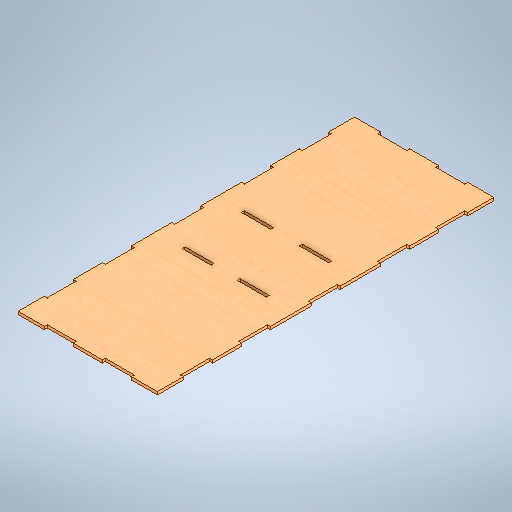
# Autodesk Inventor part: Base
Saved by Autodesk Inventor 2025 (Build 290162000, 162)
## iProperties
Created: 2024-11-02
Part Number: Base
Material: Wood (Cherry)
Document SubType Name: Sheet Metal
Designer: g.marin
Density: 0.63 g/cm^3
Sheet Metal Rule: Default
Appearance: Cherry - Natural Low Gloss
Author: g.marin
Autodesk Inventor part; units mm, degrees
ref_plane "YZ Plane" through (0, 0, 0) normal (1, 0, 0) x (0, 1, 0)
ref_plane "XZ Plane" through (0, 0, 0) normal (0, 1, 0) x (-1, 0, 0)
ref_plane "XY Plane" through (0, 0, 0) normal (0, 0, 1) x (1, 0, 0)
sketch "Sketch1" plane through (0, 0, 0) normal (0, 1, 0) x (-1, 0, 0)
  line L0 (240, 340) -> (0, 340)
  line L1 (0, 340) -> (0, 100)
  line L2 (0, 100) -> (240, 100)
  line L3 (240, 100) -> (240, 340)
  line L4 (240, 0) -> (0, 0)
  line L5 (0, 0) -> (0, -240)
  line L6 (0, -240) -> (240, -240)
  line L7 (240, -240) -> (240, 0)
  line L8 (240, 100) -> (0, 100)
  line L9 (0, 100) -> (0, 0)
  line L10 (0, 0) -> (240, 0)
  line L11 (240, 0) -> (240, 100)
  line L12 (240, 25) -> (235, 25)
  line L13 (235, 25) -> (235, 75)
  line L14 (235, 75) -> (240, 75)
  line L15 (240, 75) -> (240, 25)
  line L16 (240, 145) -> (235, 145)
  line L17 (235, 145) -> (235, 195)
  line L18 (235, 195) -> (240, 195)
  line L19 (240, 195) -> (240, 145)
  line L20 (240, 245) -> (235, 245)
  line L21 (235, 245) -> (235, 295)
  line L22 (235, 295) -> (240, 295)
  line L23 (240, 295) -> (240, 245)
  line L24 (120, -240) -> (120, 340) construction
  line L25 (240, 50) -> (0, 50) construction
  line L26 (240, -45) -> (235, -45)
  line L27 (235, -45) -> (235, -95)
  line L28 (235, -95) -> (240, -95)
  line L29 (240, -145) -> (235, -145)
  line L30 (235, -145) -> (235, -195)
  line L31 (235, -195) -> (240, -195)
  line L32 (0, 25) -> (5, 25)
  line L33 (5, 25) -> (5, 75)
  line L34 (5, 75) -> (0, 75)
  line L35 (0, 145) -> (5, 145)
  line L36 (5, 145) -> (5, 195)
  line L37 (5, 195) -> (0, 195)
  line L38 (0, 245) -> (5, 245)
  line L39 (5, 245) -> (5, 295)
  line L40 (5, 295) -> (0, 295)
  line L41 (5, -45) -> (5, -95)
  line L42 (5, -95) -> (0, -95)
  line L43 (0, -45) -> (5, -45)
  line L44 (5, -195) -> (0, -195)
  line L45 (5, -145) -> (5, -195)
  line L46 (0, -145) -> (5, -145)
  line L47 (195, -240) -> (145, -240)
  line L48 (145, -240) -> (145, -235)
  line L49 (145, -235) -> (195, -235)
  line L50 (195, -235) -> (195, -240)
  line L51 (95, -240) -> (45, -240)
  line L52 (45, -240) -> (45, -235)
  line L53 (45, -235) -> (95, -235)
  line L54 (95, -235) -> (95, -240)
  line L55 (145, 340) -> (145, 335)
  line L56 (145, 335) -> (195, 335)
  line L57 (195, 335) -> (195, 340)
  line L58 (45, 340) -> (45, 335)
  line L59 (45, 335) -> (95, 335)
  line L60 (95, 335) -> (95, 340)
  line L61 (240, -120) -> (0, -120) construction
  line L62 (240, 220) -> (0, 220) construction
  line L63 (145, 0) -> (145, -5)
  line L64 (145, -5) -> (195, -5)
  line L65 (195, -5) -> (195, 0)
  line L66 (45, 0) -> (45, -5)
  line L67 (45, -5) -> (95, -5)
  line L68 (95, -5) -> (95, 0)
  line L69 (192.5, 100) -> (142.5, 100)
  line L70 (142.5, 100) -> (142.5, 105)
  line L71 (142.5, 105) -> (192.5, 105)
  line L72 (192.5, 105) -> (192.5, 100)
  line L73 (97.5, 100) -> (47.5, 100)
  line L74 (47.5, 100) -> (47.5, 105)
  line L75 (47.5, 105) -> (97.5, 105)
  line L76 (97.5, 105) -> (97.5, 100)
  point P0 (240, 0)
  point P1 (237.5, 245)
  point P2 (240, 195)
  point P3 (240, 295)
  point P4 (195, 340)
  point P5 (145, 340)
  point P6 (95, 340)
  point P7 (45, 340)
  point P8 (0, 295)
  point P9 (0, 245)
  point P10 (0, 195)
  point P11 (0, 145)
  point P12 (0, -45)
  point P13 (0, -95)
  point P14 (0, -145)
  point P15 (0, -195)
  point P16 (45, -240)
  point P17 (145, -240)
  point P18 (240, -195)
  point P19 (240, -145)
  point P20 (240, -95)
  point P21 (240, -45)
  point P22 (145, 0)
  point P23 (195, 0)
  point P24 (45, 0)
  point P25 (95, 0)
  point P26 (97.5, 102.5)
  point P27 (142.5, 102.5)
  point P28 (120, 100)
  point P29 (47.5, 100)
  point P30 (97.5, 100)
  point P31 (192.5, 100)
  dimension "d0" = 240
  dimension "d1" = 240
  dimension "d2" = 240
  dimension "d3" = 100
  dimension "d6" = 50
  dimension "d7" = 50
  dimension "d8" = 50
  dimension "d9" = 50
  dimension "d10" = 45
  dimension "d12" = 5
  dimension "d13" = 25
  dimension "d14" = 5
  dimension "d15" = 45
  dimension "d16" = 50
  dimension "d17" = 50
  dimension "d18" = 50
  dimension "d19" = 50
  dimension "d20" = 50
  dimension "d21" = 5
  dimension "d22" = 45
  dimension "d23" = 22.5
  constraints: 154 end point, 44 symmetric about line, 20 parallel, 19 point on line, 12 midpoint, 11 perpendicular, 10 horizontal, 1 coincident
  measures "d0" distance of L2.end L0.start
  measures "d1" distance of L0.start L0.end
  measures "d2" distance of L6.end L4.start
  measures "d3" distance of L10.end L2.end
  measures "d6" distance of L12.end L13.end
  measures "d7" distance of L16.end L17.end
  measures "d8" distance of L20.end L21.end
  measures "d9" distance from line of point (237.5, 245) L18
  measures "d10" distance between parallel lines of L0 L22
  measures "d12" distance between parallel lines of L13 L15
  measures "d13" distance between parallel lines of L12 L4
  measures "d14" distance between parallel lines of L49 L6
  measures "d15" distance between parallel lines of L50 L7
  measures "d16" distance of L48.end L49.end
  measures "d17" distance of L52.end L53.end
  measures "d18" distance between parallel lines of L54 L48
  measures "d19" distance of L70.end L71.end
  measures "d20" distance of L74.end L75.end
  measures "d21" distance of L69.end L70.end
  measures "d22" distance of point (97.5, 102.5) point (142.5, 102.5)
  measures "d23" horizontal distance of point (120, 100) L70.end
extrude "Extrusion1" add sketch "Sketch1" along normal blind 5 contours L3 L22 L21 L20 L18 L17 L16 L2 L72 L71 L70 L76 L75 L74 L1 L35 L36 L37 L38 L39 L40 L0 L58 L59 L60 L55 L56 L57 | L11 L14 L13 L12 L4 L9 L32 L33 L34 L2 | L7 L26 L27 L28 L29 L30 L31 L6 L50 L49 L48 L54 L53 L52 L5 L44 L45 L46 L42 L41 L43 L4 L66 L67 L68 L63 L64 L65
equation "\"BendRadius\" = Thickness"
equation "\"BendReliefWidth\" = Thickness"
equation "\"BendReliefDepth\" = 0.5 * Thickness"
equation "\"CornerReliefSize\" = 4 * Thickness"
equation "\"MinimumRemnant\" = 2 * Thickness"
equation "\"TransitionRadius\" = BendRadius"
equation "\"JacobiRadiusSize\" = BendRadius"
equation "\"GapSize\" = Thickness"
equation "\"Thickness\" = 3.048"
body "Solid1"
